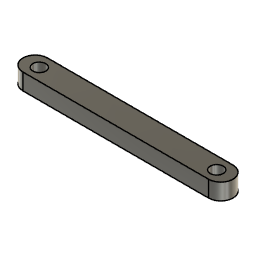
fixer_2 (Autodesk Fusion 360 design; units mm, degrees)
Autodesk Fusion 360 part; units mm, degrees
sketch "Esboço1" plane through (0, 0, 0) normal (0, 0, 1) x (1, 0, 0)
  line L0 (16.7794, 7) -> (68.3114, 7)
  line L1 (68.3114, 7) -> (68.3114, 13)
  line L2 (68.3114, 13) -> (16.7794, 13)
  line L3 (16.7794, 13) -> (16.7794, 7)
  circle A0 centre (20.7794, 10) radius 1.6
  circle A1 centre (64.3114, 10) radius 1.6
  dimension "d1" = 3.2
  dimension "d2" = 3.2
  dimension "d3" = 43.532
  dimension "d4" = 4
  dimension "d6" = 6
  dimension "d7" = 3
  dimension "d14" = 4
  constraint horizontal L0
  constraint vertical L1
  constraint horizontal L2
  constraint vertical L3
  measures "d1" diameter of A0
  measures "d2" diameter of A1
  measures "d3" distance of A0.centre A1.centre
  measures "d4" distance of L3 A0.centre
  measures "d6" distance of L0.start L2.end
  measures "d7" distance of L0 A0.centre
  measures "d14" distance of L1 A1.centre
extrude "Extrusão1" add sketch "Esboço1" along normal blind 4 makes body 1
fillet "Arredondamento1" radius 3 2 edges at (16.7794, 13, 2) (16.7794, 7, 2) on bodies 1
fillet "Arredondamento2" radius 3 2 edges at (68.3114, 13, 2) (68.3114, 7, 2) on bodies 1
copy_body "Corpo -> Componente1" bodies 1 removing the originals makes body 2 in component "Component"
scale "Escala1" factor 0.7 about (65.3114, 13, 4) bodies 2 in component "Component"
scale "Escala2" factor 1.14 about (33.439, 8.8, 1.2) bodies 2 in component "Component"
component "Component" placed x (1, 0, 0) y (0, 1, 0) z (0, 0, 1) at (0, 0, 0)
